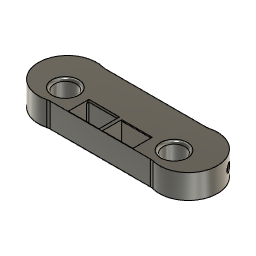
controle v1 (Autodesk Fusion 360 design; units mm, degrees)
Autodesk Fusion 360 part; units mm, degrees
sketch "Esboço1" plane through (0, 0, 0) normal (0, 0, 1) x (1, 0, 0)
  line L0 (-62.225575, 34.431563) -> (0, 34.431563)
  line L1 (-62.225575, -34.431563) -> (0, -34.431563)
  arc A0 (-65.978674, 34.908676) -> (-65.978674, -34.908676) centre (-75, 0) ccw
  circle A1 centre (-67.436181, -10.326165) radius 13.626461
  line L2 (-40, -10) -> (-2.107381, -10)
  line L3 (-2.107381, -10) -> (-2.107381, -32.453662)
  line L4 (-2.107381, -32.453662) -> (-40, -32.453662)
  line L5 (-40, -32.453662) -> (-40, -10)
  arc A2 (-62.225575, -34.431563) -> (-65.978674, -34.908676) centre (-62.225575, -49.431563) ccw
  arc A3 (-65.978674, 34.908676) -> (-62.225575, 34.431563) centre (-62.225575, 49.431563) ccw
  arc A4 (65.978674, -34.908676) -> (62.225575, -34.431563) centre (62.225575, -49.431563) ccw
  line L6 (62.225575, 34.431563) -> (0, 34.431563)
  arc A5 (65.978674, -34.908676) -> (65.978674, 34.908676) centre (75, 0) ccw
  arc A6 (62.225575, 34.431563) -> (65.978674, 34.908676) centre (62.225575, 49.431563) ccw
  line L7 (62.225575, -34.431563) -> (0, -34.431563)
  circle A7 centre (67.436181, -10.326165) radius 13.626461
  line L8 (2.107381, -32.453662) -> (40, -32.453662)
  line L9 (40, -10) -> (2.107381, -10)
  line L10 (2.107381, -10) -> (2.107381, -32.453662)
  line L11 (40, -32.453662) -> (40, -10)
  dimension "d1" = 15
  dimension "d2" = 15
  constraint horizontal L0
  constraint horizontal L1
  constraint horizontal L2
  constraint vertical L3
  constraint horizontal L4
  constraint vertical L5
  constraint tangent L1 A2
  constraint tangent A0 A2
  constraint tangent L0 A3
  constraint tangent A0 A3
  measures "d1" radius of A2
  measures "d2" radius of A3
extrude "Extrusão1" add sketch "Esboço1" along normal blind 30
fillet "Arredondamento1" radius 3 1 edges at (-80.140503, -5.398627, 30)
fillet "Arredondamento2" radius 3 1 edges at (54.731859, -5.398627, 30)
shell "Casca1" thickness 1.5 removed faces 1 at (27.369127, -10, 20)
chamfer "Chanfro1" distance 1.5 angle 45 1 faces at (-27.369127, -10, 20)
chamfer "Chanfro2" distance 1.5 angle 45 1 faces at (14.738254, -32.453662, 20)
chamfer "Chanfro3" distance 1.5 angle 45 1 faces at (-14.738254, -32.453662, 20)
sketch "Esboço2" plane through (0, 0, 0) normal (1, 0, 0) x (0, 1, 0)
  circle A0 centre (20, 15) radius 5
extrude "Extrusão2" cut sketch "Esboço2" along normal mid plane 228
